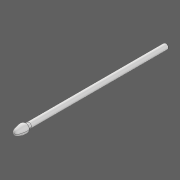
# Autodesk Inventor part: SealantApplicator
Saved by Autodesk Inventor 2020 (Build 240168000, 168)
## iProperties
Created: 2020-01-15
Part Number: SealantApplicator
Material: Generic
Document SubType Name: Modeling
Designer: Isaac Newcomb
Density: 1 g/cm^3
Appearance: Default
Author: Isaac Newcomb
Autodesk Inventor part; units mm, degrees
ref_plane "YZ Plane" through (0, 0, 0) normal (1, 0, 0) x (0, 1, 0)
ref_plane "XZ Plane" through (0, 0, 0) normal (0, 1, 0) x (-1, 0, 0)
ref_plane "XY Plane" through (0, 0, 0) normal (0, 0, 1) x (1, 0, 0)
sketch "Sketch1" plane through (0, 0, 0) normal (0, 1, 0) x (-1, 0, 0)
  line L0 (-3, -15) -> (-3, -180)
  line L1 (-3, -180) -> (0, -180)
  line L2 (0, -180) -> (0, 0)
  line L3 (0, 0) -> (-5, 0) construction
  line L4 (-7.7944, -11) -> (-3, -15) construction
  spline S0 degree 4 poles (0, 0) (-5, 0) (-2.5, -6) (-7.7944, -11) (-3, -15) knots 1 1 1 1 1 2 2 2 2 2
  line L5 (-5, 0) -> (-2.5, -6) construction
  line L6 (-2.5, -6) -> (-7.7944, -11) construction
  line L7 (-5, -10.5297) -> (0, -10.5297) construction
  line L8 (-5, -10.5297) -> (-5, -14.3364) construction
  dimension "d2" = 15
  dimension "d5" = 180
  dimension "d6" = 4
  dimension "d8" = 5
  dimension "d9" = 6
  dimension "d10" = 5
  dimension "d11" = 5
  dimension "d12" = 6
  constraints: 11 end point, 3 vertical, 2 horizontal, 2 perpendicular, 1 point on line, 4 other
  measures "d2" vertical distance of L0.start L2.end
  measures "d5" distance of L1.end L2.end
  measures "d6" vertical distance of L4.start L0.start
  measures "d8" distance of L7.start L7.end
  measures "d9" vertical distance of L3.end L5.end
  measures "d10" diameter of L5.end L2
  measures "d11" distance of L2.end L3.end
  measures "d12" diameter of L0 L2
revolve "Revolution1" add sketch "Sketch1" angle 360 about axis through (0, 0, -180) along (0, 0, 1)
fillet "Fillet1" radius 7 1 edges at (-3, 0, -15)
body "Solid1"
